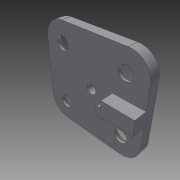
# Autodesk Inventor part: top
Saved by Autodesk Inventor 2014 (Build 180170000, 170)
## iProperties
Created: 2016-03-14
Part Number: top
Material: Generic
Document SubType Name: Modeling
Designer: buben
Density: 1 g/cm^3
Appearance: Default
Author: buben
Autodesk Inventor part; units mm, degrees
ref_plane "YZ Plane" through (0, 0, 0) normal (1, 0, 0) x (0, 1, 0)
ref_plane "XZ Plane" through (0, 0, 0) normal (0, 1, 0) x (-1, 0, 0)
ref_plane "XY Plane" through (0, 0, 0) normal (0, 0, 1) x (1, 0, 0)
sketch "Sketch1" plane through (0, 0, 0) normal (0, 1, 0) x (-1, 0, 0)
  line L0 (0, 0) -> (-32, 0)
  line L1 (-32, 0) -> (-32, -30)
  line L2 (-32, -30) -> (0, -30)
  line L3 (0, -30) -> (0, 0)
  dimension "d0" = 30
  dimension "d1" = 32
  constraints: 8 end point, 2 parallel, 1 horizontal, 1 perpendicular
  measures "d0" distance of L2.end L0.start
  measures "d1" distance of L0.start L0.end
extrude "Extrusion1" add sketch "Sketch1" along normal blind 3
sketch "Sketch2" plane through (0, 3, 0) normal (0, 1, 0) x (1, 0, 0)
  line L0 (32, 30) -> (0, 30) projected
  line L1 (0, 30) -> (0, 0) projected
  line L2 (6, 24) -> (26, 24) construction
  line L3 (26, 24) -> (26, 6) construction
  line L4 (26, 6) -> (6, 6) construction
  line L5 (6, 6) -> (6, 24) construction
  point P0 (0, 15)
  point P1 (6, 15)
  point P2 (16, 24)
  point P3 (16, 30)
  dimension "d4" = 20
  dimension "d5" = 18
  constraints: 8 end point, 4 coincident, 4 midpoint, 2 parallel, 1 horizontal, 1 horizontal alignment, 1 perpendicular, 1 vertical alignment
  measures "d4" distance of L2.start L2.end
  measures "d5" distance of L4.end L2.start
hole "Hole1" at (6, 3, -24) at (6, 3, -6) at (26, 3, -6) at (26, 3, -24) direction (0, -1, 0) diameter 4 end through all countersink diameter 8.5 countersink angle 90
sketch "Sketch3" plane through (0, 0, 0) normal (0, -1, 0) x (1, 0, 0)
  line L0 (32, 0) -> (32, -30) projected
  line L1 (32, -12.75) -> (22.75, -12.75)
  line L2 (22.75, -12.75) -> (22.75, -17.25)
  line L3 (22.75, -17.25) -> (32, -17.25)
  line L4 (32, -17.25) -> (32, -12.75)
  point P0 (32, -15)
  point P1 (32, -15)
  dimension "d13" = 9.25
  dimension "d14" = 4.5
  constraints: 8 end point, 2 midpoint, 2 parallel, 1 coincident, 1 horizontal, 1 perpendicular, 1 point on line
  measures "d13" distance of L1.start L1.end
  measures "d14" distance of L1.end L2.end
extrude "Extrusion2" add sketch "Sketch3" along normal blind 3.9
sketch "Sketch4" plane through (0, 3, 0) normal (0, 1, 0) x (1, 0, 0)
  line L0 (32, 30) -> (0, 30) projected
  line L1 (0, 30) -> (0, 0) projected
  point P0 (16, 15)
  point P1 (0, 15)
  point P2 (16, 30)
  constraints: 2 midpoint, 1 horizontal alignment, 1 vertical alignment
hole "Hole2" at (16, 3, -15) direction (0, -1, 0) diameter 3 end through all
sketch "Sketch5" plane through (0, 0, 0) normal (0, -1, 0) x (1, 0, 0)
  line L0 (0, 0) -> (32, 0) projected
  line L1 (0, -30) -> (0, 0) projected
  line L2 (9.25, -9.5) -> (22.75, -9.5) construction
  line L3 (22.75, -9.5) -> (22.75, -20.5) construction
  line L4 (22.75, -20.5) -> (9.25, -20.5) construction
  line L5 (9.25, -20.5) -> (9.25, -9.5) construction
  circle A0 centre (20.8, -18.55) radius 1.75
  point P0 (9.25, -15)
  point P1 (0, -15)
  point P2 (16, -9.5)
  point P3 (16, 0)
  dimension "d25" = 11
  dimension "d26" = 13.5
  dimension "d27" = 3.5
  dimension "d28" = 1.95
  dimension "d29" = 1.95
  constraints: 8 end point, 4 midpoint, 2 parallel, 1 centre point, 1 horizontal, 1 horizontal alignment, 1 perpendicular, 1 vertical alignment
  measures "d25" distance of L4.end L2.start
  measures "d26" distance of L2.start L2.end
  measures "d27" diameter of A0
  measures "d28" distance from line of L4 A0.centre
  measures "d29" distance from line of L3 A0.centre
extrude "Extrusion3" add sketch "Sketch5" along normal blind 2
fillet "Fillet2" radius 6 4 edges at (0, 1.5, 0) (32, 1.5, 0) (0, 1.5, -30) (32, 1.5, -30)
equation "\"d29\" = d28"
body "Solid1"
